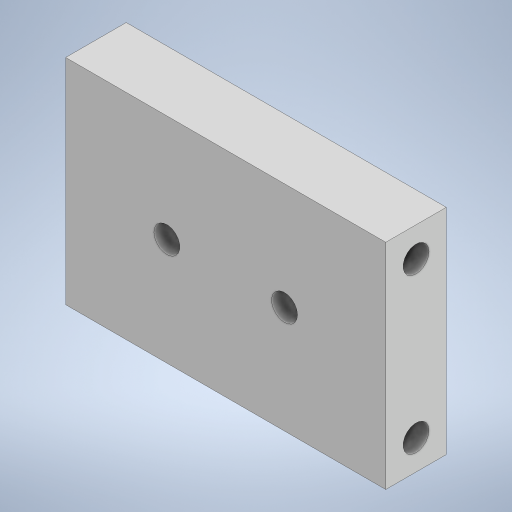
# Autodesk Inventor part: Mold_BackWall
Saved by Autodesk Inventor 2024 (Build 280153000, 153)
## iProperties
Created: 2024-09-10
Part Number: Mold_BackWall
Material: Generic
Document SubType Name: Modeling
Designer: Bruger
Density: 1 g/cm^3
Appearance: Default
Author: Bruger
Autodesk Inventor part; units mm, degrees
ref_plane "YZ Plane" through (0, 0, 0) normal (1, 0, 0) x (0, 1, 0)
ref_plane "XZ Plane" through (0, 0, 0) normal (0, 1, 0) x (-1, 0, 0)
ref_plane "XY Plane" through (0, 0, 0) normal (0, 0, 1) x (1, 0, 0)
sketch "Sketch1" plane through (0, 0, 0) normal (0, 0, 1) x (1, 0, 0)
  line L0 (-18.5, -12.375) -> (18.5, -12.375)
  line L1 (18.5, -12.375) -> (18.5, 12.375)
  line L2 (18.5, 12.375) -> (-18.5, 12.375)
  line L3 (-18.5, 12.375) -> (-18.5, -12.375)
  line L4 (-18.5, -12.375) -> (18.5, 12.375) construction
  line L5 (18.5, -12.375) -> (-18.5, 12.375) construction
  point P0 (0, 0)
  dimension "d0" = 37
  dimension "d1" = 24.75
  constraints: 12 end point, 2 midpoint, 2 parallel, 1 horizontal, 1 perpendicular
  measures "d0" distance of L2.end L1.end
  measures "d1" distance of L1.end L0.end
extrude "Extrusion1" add sketch "Sketch1" along normal blind 7
sketch "Sketch2" plane through (18.5, -12.375, 0) normal (1, 0, 0) x (0, 0, -1)
  circle A0 centre (-3.5, 3.425) radius 1.5
  line L0 (-7, 0) -> (-7, 24.75) projected
  line L1 (0, 0) -> (-7, 0) projected
  point P0 (0, 12.375)
  point P1 (-3.5, 0)
  dimension "d4" = 3
  dimension "d5" = 3.5
  dimension "d6" = 3.425
  constraints: 1 centre point, 1 midpoint
  measures "d4" diameter of A0
  measures "d5" distance from line of L0 A0.centre
  measures "d6" distance of point (-3.5, 0) A0.centre
hole "Hole1" at (18.5, -8.95, 3.5) direction (-1, 0, 0) diameter 3 depth 5 tip angle 118
mirror "Mirror1" about plane through (0, 0, 0) normal (0, 1, 0) of "Hole1"
mirror "Mirror2" about plane through (0, 0, 0) normal (1, 0, 0) of "Hole1", "Mirror1"
sketch "Sketch3" plane through (0, 0, 7) normal (0, 0, 1) x (1, 0, 0)
  circle A0 centre (6.8, 0) radius 1.5
  line L0 (18.5, 12.375) -> (-18.5, 12.375) projected
  line L1 (18.5, -12.375) -> (18.5, 12.375) projected
  point P0 (0, 0)
  dimension "d14" = 3
  dimension "d15" = 12.375
  dimension "d16" = 11.7
  constraints: 1 centre point
  measures "d14" diameter of A0
  measures "d15" distance from line of L0 A0.centre
  measures "d16" distance from line of L1 A0.centre
hole "Hole2" at (6.8, 0, 7) direction (0, 0, -1) diameter 3 end through all
mirror "Mirror3" about plane through (0, 0, 0) normal (1, 0, 0) of "Hole2"
sketch "Sketch4" plane through (-18.5, -12.375, 0) normal (0, -1, 0) x (1, 0, 0)
  circle A0 centre (18.9, 3.5) radius 1.5
  line L0 (0, 7) -> (37, 7) projected
  line L1 (0, 0) -> (0, 7) projected
  point P0 (18.5, 0)
  dimension "d24" = 3
  dimension "d25" = 3.5
  dimension "d26" = 18.9
  constraints: 1 centre point
  measures "d24" diameter of A0
  measures "d25" distance from line of L0 A0.centre
  measures "d26" distance from line of L1 A0.centre
hole "Hole3" at (0.4, -12.375, 3.5) direction (0, 1, 0) diameter 3 depth 5 tip angle 118
body "Solid1"
